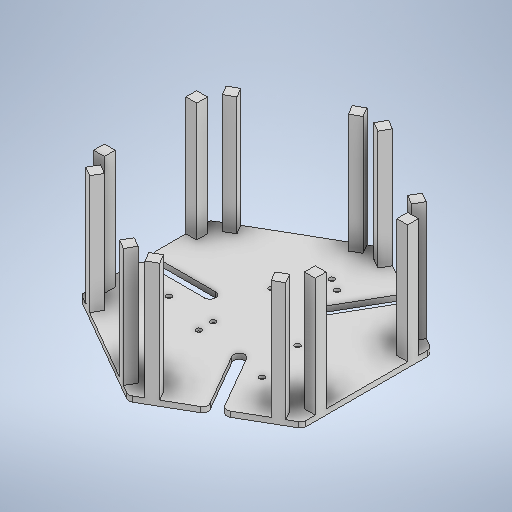
# Autodesk Inventor part: RT_FRM_MC_011_TB_TopPlate
Saved by Autodesk Inventor 2025.4 (Build 294407000, 407)
## iProperties
Created: 2026-04-28
Part Number: RT_FRM_MC_011_TB_TopPlate
Material: Generic
Document SubType Name: Modeling
Designer: louis
Density: 1 g/cm^3
Appearance: Default
Mass: 556.266 g
Surface Area: 1307.88 cm^2
Volume: 556.266 cm^3
Author: louis
Autodesk Inventor part; units mm, degrees
ref_plane "YZ Plane" through (0, 0, 0) normal (1, 0, 0) x (0, 1, 0)
ref_plane "XZ Plane" through (0, 0, 0) normal (0, 1, 0) x (-1, 0, 0)
ref_plane "XY Plane" through (0, 0, 0) normal (0, 0, 1) x (1, 0, 0)
sketch "Sketch1" plane through (0, 0, 0) normal (0, 1, 0) x (-1, 0, 0)
  line L0 (25, -2.5) -> (135, -2.5)
  line L1 (135, 0) -> (25, 0)
  line L2 (0, 0) -> (25, 0)
  circle A0 centre (0, 0) radius 237.5 construction
  line L3 (50, 0) -> (103.8137, 0) construction
  line L4 (130, 26.5) -> (30, 26.5)
  line L5 (30, 26.5) -> (30, 76.5)
  line L6 (30, 76.5) -> (130, 76.5)
  line L7 (130, 76.5) -> (130, 26.5)
  line L8 (80, 26.5) -> (80, 0) construction
  line L9 (80, 76.5) -> (80, 26.5) construction
  line L10 (121, 40.5) -> (80, 40.5) construction
  line L11 (121, 40.5) -> (121, 67) construction
  line L12 (237.2894, -10) -> (75, -10)
  line L13 (75, -10) -> (75, 10)
  line L14 (75, 10) -> (237.2894, 10)
  line L15 (237.2894, 10) -> (237.2894, -10)
  line L16 (0, 0) -> (0, 237.5)
  line L17 (155, 10) -> (155, 110)
  line L18 (155, 110) -> (-63.5085, 110)
  line L19 (-63.5085, 110) -> (0, 0)
  circle A1 centre (0, 0) radius 300 construction
  line L20 (-300, -380) -> (-300, -300) construction
  line L21 (-300, -300) -> (-380, -300) construction
  line L22 (-380, -300) -> (-380, -380) construction
  line L23 (-380, -380) -> (-300, -380) construction
  line L24 (-300, -380) -> (-380, -300) construction
  line L25 (-300, -300) -> (-380, -380) construction
  line L26 (-300, 300) -> (-300, 380) construction
  line L27 (-300, 380) -> (-380, 380) construction
  line L28 (-380, 380) -> (-380, 300) construction
  line L29 (-380, 300) -> (-300, 300) construction
  line L30 (-300, 300) -> (-380, 380) construction
  line L31 (-300, 380) -> (-380, 300) construction
  line L32 (380, 300) -> (380, 380) construction
  line L33 (380, 380) -> (300, 380) construction
  line L34 (300, 380) -> (300, 300) construction
  line L35 (300, 300) -> (380, 300) construction
  line L36 (380, 300) -> (300, 380) construction
  line L37 (380, 380) -> (300, 300) construction
  line L38 (380, -380) -> (380, -300) construction
  line L39 (380, -300) -> (300, -300) construction
  line L40 (300, -300) -> (300, -380) construction
  line L41 (300, -380) -> (380, -380) construction
  line L42 (380, -380) -> (300, -300) construction
  line L43 (380, -300) -> (300, -380) construction
  line L44 (300, -300) -> (300, 300) construction
  line L45 (300, 300) -> (-300, 300) construction
  line L46 (-300, 300) -> (-300, -300) construction
  line L47 (-300, -300) -> (300, -300) construction
  line L48 (-205.681, -118.75) -> (-205.681, 118.75)
  line L49 (-205.681, 118.75) -> (0, 237.5)
  line L50 (0, 237.5) -> (205.681, 118.75)
  line L51 (205.681, 118.75) -> (205.681, -118.75)
  line L52 (205.681, -118.75) -> (0, -237.5)
  line L53 (0, -237.5) -> (-205.681, -118.75)
  line L54 (-63.5085, 110) -> (-102.8405, 178.125)
  point P0 (39, 40.5)
  point P1 (39, 67)
  point P2 (229.7961, -60)
  point P3 (75, 0)
  point P4 (0, 237.5)
  point P5 (0, 110)
  point P6 (205.681, 10)
  point P7 (0, 237.5)
  dimension "d0" = 110
  dimension "d2" = 2.5
  dimension "d4" = 80
  dimension "d9" = 475
  dimension "d11" = 29
  dimension "d12" = 50
  dimension "d13" = 100
  dimension "d14" = 26.5
  dimension "d15" = 82
  dimension "d26" = 20
  dimension "d27" = 5
  dimension "d33" = 9.5
  dimension "d40" = 50
  dimension "d46" = 120
  dimension "d47" = 100
  dimension "d48" = 25
  dimension "d74" = 80
  dimension "d75" = 80
  dimension "d78" = 80
  dimension "d79" = 80
  dimension "d80" = 80
  dimension "d81" = 80
  dimension "d82" = 80
  dimension "d83" = 80
  dimension "d84" = 600
  constraints: 110 end point, 14 perpendicular, 12 parallel, 8 vertical, 5 point on circle, 4 coincident, 4 horizontal, 4 midpoint, 3 point on line, 3 tangent, 2 centre point, 2 symmetric about line, 1 collinear, 13 other
  measures "d0" distance of L0.end L0.start
  measures "d2" distance between parallel lines of L0 L1
  measures "d4" distance of L2.start L8.end
  measures "d9" diameter of A0
  measures "d11" distance from line of L0 L4.start
  measures "d12" distance of L6.end L4.start
  measures "d13" distance of L4.start L4.end
  measures "d14" distance of L11.end L10.start
  measures "d15" distance of L10.start point (39, 40.5)
  measures "d26" distance between parallel lines of L14 L12
  measures "d27" distance between parallel lines of L8 L13
  measures "d33" distance from line of L6 L11.end
  measures "d40" distance from line of L12 point (229.796, -60)
  measures "d46" angle of L19 L2
  measures "d47" distance of L17.start L17.end
  measures "d48" distance between parallel lines of L17 L7
  measures "d74" distance of L21.end L22.end
  measures "d75" distance of L22.end L20.start
  measures "d78" distance of L27.end L28.end
  measures "d79" distance of L28.end L26.start
  measures "d80" distance of L33.end L34.end
  measures "d81" distance of L34.end L32.start
  measures "d82" distance of L39.end L40.end
  measures "d83" distance of L40.end L38.start
  measures "d84" diameter of A1
extrude "Extrusion1" add sketch "Sketch1" against normal blind 10 contours L1 L2 L16 L18 L17 L14 L13 | L19 L18 L16 | L17 L18 L16 L50 L51 L14 | L18 L54 L49 L16 | L4 L5 L6 L7
pattern_circular "Circular Pattern2" count 3 over 360 about axis through (0, 0, 0) along (0, -1, 0) of "Extrusion1"
hole "Hole1" at (-121, 0, 40.5) at (-39, 0, 40.5) at (-121, 0, 67) at (-39, 0, 67) direction (0, -1, 0) diameter 5.5 end through all counterbore diameter 10 counterbore depth 5 clearance for "Socket Head Cap Screw" size "M5" standard "Ansi Metric M Profile"
extrude "Extrusion2" cut sketch "Sketch1" against normal blind 10 contours L13 L14 L51 L12 | L51 L14 L15 L12
pattern_circular "Circular Pattern1" count 3 over 360 about axis through (0, -10, 0) along (0, 1, 0) of "Hole1", "Extrusion2"
fillet "Fillet1" radius 10 18 edges at (28.8397, -5, 69.9519) (46.1603, -5, -59.9519) (-75, -5, -10) (-75, -5, 10) (46.1603, -5, 59.9519) (28.8397, -5, -69.9519) (0, -5, -237.5) (205.681, -5, -118.75) (111.5008, -5, -173.125) (94.1803, -5, -183.125) (111.5008, -5, 173.125) (94.1803, -5, 183.125) (-205.681, -5, 10) (-205.681, -5, -10) (-205.681, -5, -118.75) (205.681, -5, 118.75) (0, -5, 237.5) (-205.681, -5, 118.75)
sketch "Sketch2" plane through (0, -10, 0) normal (0, 1, 0) x (1, 0, 0)
  line L0 (-85, 0) -> (0, 0) construction
  line L1 (0, 0) -> (0, 200) construction
  line L2 (-20, 0) -> (-20, 20) construction
  line L3 (-20, 20) -> (20, 20) construction
  line L4 (20, 20) -> (20, 0) construction
  line L5 (20, 0) -> (-20, 0) construction
  arc A0 (-85, -10) -> (-85, 10) centre (-85, 0) ccw projected
  line L6 (-20, -20) -> (-20, -100) construction
  line L7 (-20, -100) -> (20, -100) construction
  line L8 (20, 0) -> (20, -102.2687) construction
  point P0 (-20, 150)
  point P1 (20, 150)
  point P2 (-70, 10)
  point P3 (-70, -10)
  point P4 (-60, 0)
  point P5 (20, -20)
  dimension "d52" = 90
  dimension "d53" = 200
  dimension "d54" = 40
  dimension "d55" = 20
  dimension "d58" = 130
  dimension "d85" = 80
  constraints: 18 end point, 5 perpendicular, 3 coincident, 3 symmetric about line, 2 point on line, 2 vertical, 1 horizontal, 1 parallel, 2 other
  measures "d52" angle of L0 L1
  measures "d53" distance of L0.end L1.end
  measures "d54" distance of L4.end L2.start
  measures "d55" distance of L3.end L4.end
  measures "d58" distance of point (-20, 20) point (-20, 150)
  measures "d85" distance of L6.start L6.end
hole "Hole2" [suppressed]
sketch "Sketch3" plane through (0, 0, 0) normal (0, 1, 0) x (1, 0, 0)
  line L0 (120.161, -168.125) -> (200.681, -121.6368) projected
  line L1 (185.681, -130.297) -> (168.3605, -140.297)
  line L2 (168.3605, -140.297) -> (158.3605, -122.9765)
  line L3 (158.3605, -122.9765) -> (175.681, -112.9765)
  line L4 (175.681, -112.9765) -> (185.681, -130.297)
  line L5 (205.681, -112.9765) -> (205.681, 112.9765) projected
  line L6 (205.681, -95.656) -> (205.681, -75.656)
  line L7 (205.681, -75.656) -> (185.681, -75.656)
  line L8 (185.681, -75.656) -> (185.681, -95.656)
  line L9 (185.681, -95.656) -> (205.681, -95.656)
  line L10 (205.681, -112.9765) -> (185.681, -95.656) construction
  line L11 (200.681, -121.6368) -> (175.681, -112.9765) construction
  point P0 (0, 0)
  dimension "d86" = 20
  dimension "d90" = 20
  dimension "d91" = 20
  dimension "d92" = 20
  dimension "d93" = 20
  constraints: 20 end point, 4 parallel, 4 point on line, 2 perpendicular, 1 equal length
  measures "d86" distance of L1.end L2.end
  measures "d90" distance of L2.end L3.end
  measures "d91" distance of L6.start L6.end
  measures "d92" distance of L7.end L6.end
  measures "d93" distance of L3.end L8.end
extrude "Extrusion3" add sketch "Sketch3" along normal blind 220
pattern_circular "Circular Pattern4" count 6 over 360 about axis through (0, -10, 0) along (0, 1, 0) of "Extrusion3"
body "Solid1"
